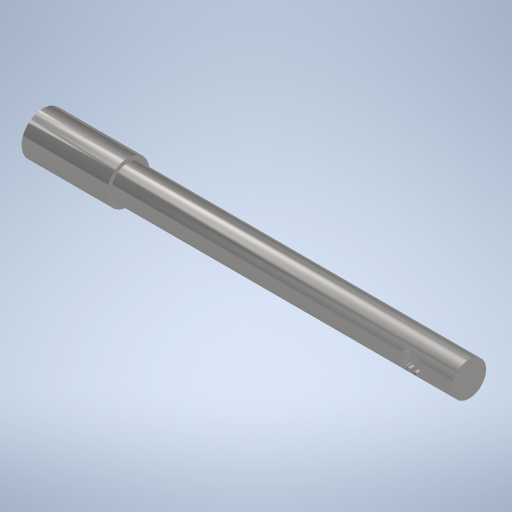
# Autodesk Inventor part: 4x2020_axis
Saved by Autodesk Inventor 2024 (Build 280153000, 153)
## iProperties
Created: 2025-12-17
Part Number: 4x2020_axis
Material: Stainless Steel
Document SubType Name: Modeling
Designer: schar
Density: 8 g/cm^3
Appearance: Semi-Polished
Author: schar
Autodesk Inventor part; units mm, degrees
ref_plane "YZ Plane" through (0, 0, 0) normal (1, 0, 0) x (0, 1, 0)
ref_plane "XZ Plane" through (0, 0, 0) normal (0, 1, 0) x (-1, 0, 0)
ref_plane "XY Plane" through (0, 0, 0) normal (0, 0, 1) x (1, 0, 0)
sketch "Sketch1" plane through (0, 0, 0) normal (1, 0, 0) x (0, 1, 0)
  circle A0 centre (0, 0) radius 4
  circle A1 centre (0, 0) radius 5
  dimension "d0" = 8
  dimension "d1" = 10
  constraints: 2 centre point, 2 coincident
  measures "d0" diameter of A0
  measures "d1" diameter of A1
extrude "Extrusion1" add sketch "Sketch1" along normal blind 20
ref_plane "Work Plane1" through (15, 0, 0) normal (1, 0, 0) x (0, 0, -1)
sketch "Sketch2" plane through (15, 0, 0) normal (1, 0, 0) x (0, 0, -1)
  circle A0 centre (0, 0) radius 4
  constraints: 1 centre point, 1 coincident
extrude "Extrusion2" add sketch "Sketch2" along normal blind 85
sketch "Sketch3" plane through (0, 0, 0) normal (0, 1, 0) x (-1, 0, 0)
  line L0 (0, 0) -> (-7.5, 0)
  circle A0 centre (-7.5, 0) radius 1.5
  dimension "d7" = 7.5
  dimension "d8" = 3
  constraints: 2 end point, 1 centre point, 1 coincident, 1 horizontal
  measures "d7" distance of L0.start L0.end
  measures "d8" diameter of A0
extrude "Extrusion3" cut sketch "Sketch3" against normal blind 60
thread "Thread1" size "M3x0.5" class "6H" standard "ANSI Metric M Profile" length 70
sketch "Sketch4" plane through (0, 0, 0) normal (0, 0, 1) x (1, 0, 0)
  line L0 (100, -4) -> (100, 4) projected
  line L1 (100, 0) -> (90, 0)
  circle A0 centre (90, 0) radius 2
  point P0 (0, 0)
  dimension "d13" = 10
  dimension "d14" = 4
  constraints: 2 end point, 1 centre point, 1 coincident, 1 horizontal, 1 midpoint
  measures "d13" distance of L1.start L1.end
  measures "d14" diameter of A0
extrude "Extrusion4" cut sketch "Sketch4" along normal blind 10
sketch "Sketch5" plane through (90, 0, 0) normal (0, 0, 1) x (1, 0, 0)
  circle A0 centre (0, 0) radius 2
  point P0 (-90, 0)
  constraints: 1 centre point
extrude "Extrusion5" add sketch "Sketch5" along normal blind 2
chamfer "Chamfer1" distance 0.5 angle 45 1 edges at (88.0001, -0.0148, 4)
body "Solid1"
